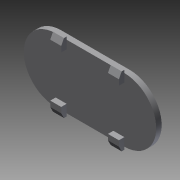
# Autodesk Inventor part: 276-2243
Saved by Autodesk Inventor 2013 (Build 170138000, 138)
## iProperties
Category: Power
Company: Autodesk Inc.
Created: 2012-02-07
Part Number: 276-2243
Document SubType Name: Modeling
Designer: Autodesk Inc.
Density: 1.06 g/cm^3
Material: ABS Plastic
Catalog Web Link: http://www.vexrobotics.com/276-2243.html
Vendor: VEX
Mass: 0.277871 g
Surface Area: 5.96791 cm^2
Volume: 0.262143 cm^3
Author: Autodesk Inc.
Autodesk Inventor part; units mm, degrees
ref_plane "YZ Plane" through (0, 0, 0) normal (1, 0, 0) x (0, 1, 0)
ref_plane "XZ Plane" through (0, 0, 0) normal (0, 1, 0) x (-1, 0, 0)
ref_plane "XY Plane" through (0, 0, 0) normal (0, 0, 1) x (1, 0, 0)
sketch "Sketch1" plane through (0, 0, 0) normal (0, 0, 1) x (1, 0, 0)
  line L0 (-6.25, -5.7997) -> (6.25, -5.7997)
  arc A0 (6.25, -5.7997) -> (6.25, 5.7997) centre (6.25, 0) ccw
  line L1 (6.25, 5.7997) -> (-6.25, 5.7997)
  arc A1 (-6.25, 5.7997) -> (-6.25, -5.7997) centre (-6.25, 0) ccw
  point P0 (0, 0)
  point P1 (0, 0)
  constraints: 4 end point, 4 point on circle, 2 centre point
extrude "Extrusion1" add sketch "Sketch1" against normal blind 0.9906
sketch "Sketch2" plane through (0, 0, 0) normal (0, 0, 1) x (1, 0, 0)
  line L0 (-6.25, 6.2997) -> (-4.25, 6.2997)
  line L1 (-6.25, 5.7997) -> (-6.25, 6.2997)
  line L2 (-4.25, 5.7997) -> (-6.25, 5.7997)
  line L3 (-4.25, 6.2997) -> (-4.25, 5.7997)
  line L4 (-6.25, 4.2997) -> (-6.25, 5.7997)
  line L5 (-4.25, 5.7997) -> (-4.25, 4.2997)
  line L6 (-4.25, 4.2997) -> (-6.25, 4.2997)
  line L7 (4.25, 6.2997) -> (6.25, 6.2997)
  line L8 (4.25, 5.7997) -> (4.25, 6.2997)
  line L9 (6.25, 6.2997) -> (6.25, 5.7997)
  line L10 (4.25, 4.2997) -> (4.25, 5.7997)
  line L11 (6.25, 5.7997) -> (6.25, 4.2997)
  line L12 (6.25, 4.2997) -> (4.25, 4.2997)
  line L13 (-4.25, -6.2997) -> (-6.25, -6.2997)
  line L14 (-4.25, -5.7997) -> (-4.25, -6.2997)
  line L15 (-6.25, -5.7997) -> (-4.25, -5.7997)
  line L16 (-6.25, -6.2997) -> (-6.25, -5.7997)
  line L17 (-6.25, -5.7997) -> (-6.25, -4.2997)
  line L18 (-6.25, -4.2997) -> (-4.25, -4.2997)
  line L19 (-4.25, -4.2997) -> (-4.25, -5.7997)
  line L20 (6.25, -5.2997) -> (6.25, -6.2997)
  line L21 (4.25, -6.2997) -> (4.25, -5.7997)
  line L22 (6.25, -6.2997) -> (4.25, -6.2997)
  line L23 (4.25, -5.7997) -> (4.25, -4.2997)
  line L24 (4.25, -4.2997) -> (6.25, -4.2997)
  line L25 (6.25, -4.2997) -> (6.25, -5.7997)
  point P0 (0, 0)
  point P1 (6.25, 0)
  point P2 (-6.25, 0)
  point P3 (0, 0)
  constraints: 52 end point
extrude "Extrusion2" add sketch "Sketch2" along normal blind 0.9906
chamfer "Chamfer1" distance 0.508 distance2 0.9906 1 edges at (-5.25, 6.2997, 0.9906) measured on face at (-4.9167, 6.2997, 0.3302)
chamfer "Chamfer2" distance 0.508 distance2 0.9906 1 edges at (5.25, 6.2997, 0.9906) measured on face at (5.5833, 6.2997, 0.3302)
chamfer "Chamfer3" distance 0.508 distance2 0.9906 1 edges at (5.25, -6.2997, 0.9906) measured on face at (4.9167, -6.2997, 0.3302)
chamfer "Chamfer4" distance 0.508 distance2 0.9906 1 edges at (-5.25, -6.2997, 0.9906) measured on face at (-5.5833, -6.2997, 0.3302)
body "Solid1"
